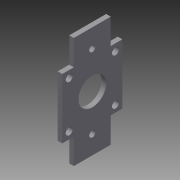
# Autodesk Inventor part: Plate
Saved by Autodesk Inventor 2014 (Build 180170000, 170)
## iProperties
Created: 2014-01-07
Part Number: Plate
Material: Generic
Document SubType Name: Modeling
Designer: Andrew Toennies
Density: 1 g/cm^3
Appearance: Default
Author: Andrew Toennies
Autodesk Inventor part; units mm, degrees
ref_plane "YZ Plane" through (0, 0, 0) normal (1, 0, 0) x (0, 1, 0)
ref_plane "XZ Plane" through (0, 0, 0) normal (0, 1, 0) x (-1, 0, 0)
ref_plane "XY Plane" through (0, 0, 0) normal (0, 0, 1) x (1, 0, 0)
sketch "Sketch1" plane through (0, 0, 0) normal (1, 0, 0) x (0, 1, 0)
  line L0 (76.2, 0) -> (76.2, -25.4)
  line L1 (0, -25.4) -> (0, 0)
  line L2 (58.7375, 7.9375) -> (17.4625, 7.9375)
  line L3 (17.4625, -33.3375) -> (58.7375, -33.3375)
  line L4 (76.2, -25.4) -> (58.7375, -25.4)
  line L5 (17.4625, -25.4) -> (0, -25.4)
  line L6 (17.4625, 7.9375) -> (17.4625, 0)
  line L7 (17.4625, -25.4) -> (17.4625, -33.3375)
  line L8 (0, 0) -> (17.4625, 0)
  line L9 (58.7375, 0) -> (76.2, 0)
  line L10 (58.7375, -33.3375) -> (58.7375, -25.4)
  line L11 (58.7375, 0) -> (58.7375, 7.9375)
  circle A0 centre (63.5, -12.7) radius 2.0828
  circle A1 centre (12.7, -12.7) radius 2.0828
  line L12 (53.975, 3.175) -> (22.225, 3.175) construction
  line L13 (22.225, 3.175) -> (22.225, -28.575) construction
  line L14 (22.225, -28.575) -> (53.975, -28.575) construction
  line L15 (53.975, -28.575) -> (53.975, 3.175) construction
  circle A2 centre (53.975, 3.175) radius 2.3876
  circle A3 centre (53.975, -28.575) radius 2.3876
  circle A4 centre (22.225, 3.175) radius 2.3876
  circle A5 centre (22.225, -28.575) radius 2.3876
  circle A6 centre (38.1, -12.7) radius 9.525
  dimension "d0" = 25.4
  dimension "d1" = 76.2
  dimension "d2" = 41.275
  dimension "d3" = 41.275
  dimension "d4" = 25.4
  dimension "d5" = 4.1656
  dimension "d6" = 4.1656
  dimension "d7" = 31.75
  dimension "d8" = 31.75
  dimension "d9" = 3.175
  dimension "d10" = 4.7625
  dimension "d11" = 12.7
  dimension "d12" = 12.7
  dimension "d13" = 12.7
  dimension "d14" = 12.7
  dimension "d15" = 4.7752
  dimension "d18" = 31.75
  dimension "d21" = 31.75
  dimension "d24" = 19.05
  dimension "d25" = 20.6375
  dimension "d26" = 20.6375
  constraints: 32 end point, 12 parallel, 7 centre point, 5 collinear, 5 horizontal, 5 perpendicular, 1 coincident, 1 vertical, 6 other
  measures "d0" distance of L0.start L0.end
  measures "d1" distance of L0.end L1.start
  measures "d2" distance of L3.start L3.end
  measures "d3" distance between parallel lines of L3 L2
  measures "d4" distance between parallel lines of L8 L5
  measures "d5" diameter of A0
  measures "d6" diameter of A1
  measures "d7" distance of L14.end L12.start
  measures "d8" distance of L13.end L14.end
  measures "d9" distance between parallel lines of L8 L12
  measures "d10" distance between parallel lines of L11 L15
  measures "d11" distance from line of L0 A0.centre
  measures "d12" distance from line of L4 A0.centre
  measures "d13" distance from line of A1.centre L1
  measures "d14" distance from line of L5 A1.centre
  measures "d15" diameter of A2
  measures "d18" distance of A2.centre A3.centre
  measures "d21" distance of A2.centre A4.centre
  measures "d24" diameter of A6
  measures "d25" distance from line of L2 A6.centre
  measures "d26" distance from line of L11 A6.centre
extrude "Extrusion1" add sketch "Sketch1" along normal blind 3.175
body "Solid1"
